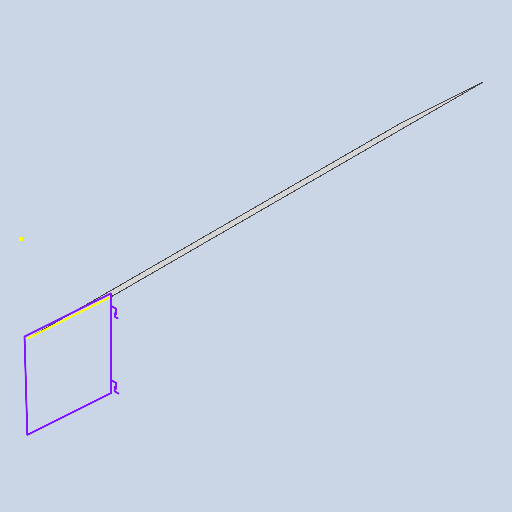
# Autodesk Inventor part: MSC 0101 sheet gills
Saved by Autodesk Inventor 2025 (Build 290162010, 162A)
## iProperties
Created: 2024-06-15
Part Number: MSC 0101 sheet gills
Material: Stainless Steel
Document SubType Name: Sheet Metal
Designer: pokla
Density: 8 g/cm^3
Sheet Metal Rule: Default_mm
Appearance: Default
Stock Number: МОО 0101 лист жабра
Mass: 10993.3 g
Surface Area: 55005.7 cm^2
Volume: 1374.16 cm^3
Author: pokla
Autodesk Inventor part; units mm, degrees
ref_plane "YZ Plane" through (0, 0, 0) normal (1, 0, 0) x (0, 1, 0)
ref_plane "XZ Plane" through (0, 0, 0) normal (0, 1, 0) x (-1, 0, 0)
ref_plane "XY Plane" through (0, 0, 0) normal (0, 0, 1) x (1, 0, 0)
sketch "Sketch1" plane through (0, 0, 0) normal (0, 0, 1) x (1, 0, 0)
  line L0 (-750, 0) -> (750, 0) construction
  line L1 (750, 0) -> (750, -2100) construction
  line L2 (750, -2100) -> (110, -2700) construction
  line L3 (110, -2700) -> (-110, -2700) construction
  line L4 (-110, -2700) -> (-750, -2100) construction
  line L5 (-750, -2100) -> (-750, 0) construction
  line L6 (-725, -40) -> (725, -40) construction
  line L7 (-725, -2089.1692) -> (-100.1138, -2675) construction
  line L8 (-100.1138, -2675) -> (100.1138, -2675) construction
  line L9 (100.1138, -2675) -> (725, -2089.1692) construction
  line L10 (0, -2700) -> (0, 0) construction
  line L11 (55, -2700) -> (55, 0) construction
  line L12 (-55, -2700) -> (-55, 0) construction
  line L13 (725, -2089.1692) -> (725, -40) construction
  line L14 (-725, -40) -> (-725, -2089.1692) construction
  line L15 (725, -40) -> (55, -664.7851)
  point P0 (0, -40)
  dimension "d0" = 1500
  dimension "d2" = 220
  dimension "d3" = 600
  dimension "d5" = 2700
  dimension "d7" = 40
  dimension "d10" = 1450
  dimension "d11" = 25
  dimension "d13" = 55
  dimension "d14" = 55
  dimension "d16" = 133
  measures "d0" distance of L0.start L0.end
  measures "d2" distance of L2.end L3.end
  measures "d3" vertical distance of L2.end L1.end
  measures "d5" distance between parallel lines of L0 L3
  measures "d7" distance between parallel lines of L0 L6
  measures "d10" distance of L6.end L6.start
  measures "d11" distance between parallel lines of L3 L8
  measures "d13" distance between parallel lines of L10 L11
  measures "d14" distance between parallel lines of L10 L12
  measures "d16" angle of L13 L15
contour flange "Contour Flange1" sketch "Sketch1" thickness 0.5 bend radius 0.5 width 3000 along (0, 0, -1) mid plane no both sides no wall seen from (390, -352.3926, 0) lies toward (0.6819984, -0.7313537, 0) curves L15
bend "Bend1"
corner "Corner1"
sketch "Sketch2" plane through (0, 0, 0) normal (0, 0, 1) x (1, 0, 0)
  line L0 (725, -14.0576) -> (725, -711.6361)
  line L1 (725, -711.6361) -> (51.2725, -1339.8971)
  line L2 (725, -40) -> (55, -664.7851) projected
  line L3 (51.2725, -1339.8971) -> (28.6081, -664.7851)
  line L4 (28.6081, -664.7851) -> (725, -15.3891)
  line L5 (725, -102) -> (764.4623, -102)
  line L6 (725, -619.8366) -> (764.4623, -619.8366)
  line L7 (764.4623, -619.8366) -> (764.4623, -664.7851)
  line L8 (764.4623, -102) -> (764.4623, -145.6915)
  line L9 (756.8069, -136.967) -> (756.8069, -162.3163)
  line L10 (756.8069, -162.3163) -> (780.2062, -162.3163)
  line L11 (754.6633, -650.9815) -> (754.6633, -683.9746)
  line L12 (754.6633, -683.9746) -> (788.2377, -683.9746)
  point P0 (0, 0)
  constraints: 24 end point, 4 vertical, 3 perpendicular, 2 horizontal, 2 parallel, 2 point on line
equation "\"d14\" = d13"
equation "\"d17\" = Thickness"
equation "\"d18\" = BendReliefWidth"
equation "\"d19\" = BendReliefDepth"
equation "\"d20\" = MinimumRemnant"
equation "\"d21\" = TransitionRadius"
equation "\"d23\" = BendRadius"
equation "\"d25\" = CornerReliefSize"
equation "\"d26\" = GapSize"
equation "\"d27\" = JacobiRadiusSize"
equation "\"BendRadius\" = Thickness"
equation "\"BendReliefWidth\" = Thickness"
equation "\"BendReliefDepth\" = 0.5 * Thickness"
equation "\"CornerReliefSize\" = 4 * Thickness"
equation "\"MinimumRemnant\" = 2 * Thickness"
equation "\"TransitionRadius\" = BendRadius"
equation "\"JacobiRadiusSize\" = BendRadius"
equation "\"GapSize\" = Thickness"
equation "\"Thickness\" = 0.5"
body "Solid1"
